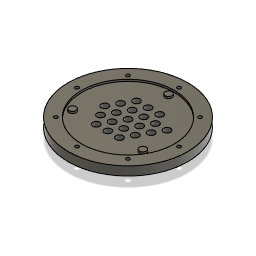
Feed.Through.Adapter (Autodesk Fusion 360 design; units mm, degrees)
Autodesk Fusion 360 part; units mm, degrees
note: some values were not read from the file. Chosen so that the rebuilt part matches the saved one: which bodies a step acts on.
sketch "Active.Area" plane through (0, 0, 0) normal (0, 1, 0) x (1, 0, 0)
  circle A0 centre (0, 0) radius 30
  circle A1 centre (0, 0) radius 40 construction
  circle A2 centre (0, -35) radius 3.175 construction
  circle A3 centre (30.3109, 17.5) radius 3.175 construction
  circle A4 centre (-30.3109, 17.5) radius 3.175 construction
  dimension "d1" = 60
  dimension "d2" = 80
  dimension "d4" = 6.35
  dimension "d6" = 360
  constraint coincident A0.centre A1.centre
  constraint concentric A0 A1
  measures "d1" diameter of A0
  measures "d2" diameter of A1
  measures "d4" diameter of A2
sketch "Feed.Through.Adapter.B" plane through (0, 0, 0) normal (0, 1, 0) x (1, 0, 0)
  circle A0 centre (0, 0) radius 34
  circle A1 centre (0, 0) radius 32 construction
  circle A2 centre (0, 32) radius 1
  circle A3 centre (-27.7128, -16) radius 1
  circle A4 centre (27.7128, -16) radius 1
  circle A5 centre (0, 0) radius 30 construction
  dimension "d7" = 68
  dimension "d8" = 64
  dimension "d9" = 2
  dimension "d11" = 360
  dimension "d12" = 60
  constraint coincident A0.centre A1.centre
  constraint concentric A0 A1
  constraint concentric A1 A5
  measures "d7" diameter of A0
  measures "d8" diameter of A1
  measures "d9" diameter of A2
  measures "d12" diameter of A5
sketch "Holes/Cuts" plane through (0, 0, 0) normal (0, 1, 0) x (1, 0, 0)
  circle A0 centre (0, 0) radius 30 construction
  circle A1 centre (0, 0) radius 3
  circle A2 centre (10, 0) radius 3
  circle A3 centre (5, 8.6603) radius 3
  circle A4 centre (-5, 8.6603) radius 3
  circle A5 centre (-10, 0) radius 3
  circle A6 centre (-5, -8.6603) radius 3
  circle A7 centre (5, -8.6603) radius 3
  circle A8 centre (15, 8.6603) radius 3
  circle A9 centre (0, 17.3205) radius 3
  circle A10 centre (-15, 8.6603) radius 3
  circle A11 centre (-15, -8.6603) radius 3
  circle A12 centre (0, -17.3205) radius 3
  circle A13 centre (15, -8.6603) radius 3
  circle A14 centre (20, 0) radius 3
  circle A15 centre (10, 17.3205) radius 3
  circle A16 centre (-10, 17.3205) radius 3
  circle A17 centre (-20, 0) radius 3
  circle A18 centre (-10, -17.3205) radius 3
  circle A19 centre (10, -17.3205) radius 3
  circle A20 centre (25, 8.6603) radius 3
  circle A21 centre (0, 0) radius 31
  circle A22 centre (0, 0) radius 40
  circle A23 centre (20, 0) radius 0.5
  circle A24 centre (10, 0) radius 0.5
  circle A25 centre (0, 0) radius 0.5
  circle A26 centre (15, -8.6603) radius 0.5
  circle A27 centre (5, 8.6603) radius 0.5
  circle A28 centre (10, 17.3205) radius 0.5
  circle A29 centre (15, 8.6603) radius 0.5
  circle A30 centre (-5, 8.6603) radius 0.5
  circle A31 centre (-10, 17.3205) radius 0.5
  circle A32 centre (0, 17.3205) radius 0.5
  circle A33 centre (-10, 0) radius 0.5
  circle A34 centre (-20, 0) radius 0.5
  circle A35 centre (-15, 8.6603) radius 0.5
  circle A36 centre (-5, -8.6603) radius 0.5
  circle A37 centre (-10, -17.3205) radius 0.5
  circle A38 centre (-15, -8.6603) radius 0.5
  circle A39 centre (5, -8.6603) radius 0.5
  circle A40 centre (10, -17.3205) radius 0.5
  circle A41 centre (0, -17.3205) radius 0.5
  circle A42 centre (25, 8.6603) radius 0.5
  dimension "d39" = 6
  dimension "d52" = 62
  dimension "d112" = 80
  dimension "d179" = 1
  dimension "d180" = 1
  dimension "d181" = 1
  dimension "d182" = 1
  dimension "d184" = 360
  dimension "d185" = 1
  constraint coincident A0.centre A1.centre
  constraint concentric A1 A22
  constraint concentric A14 A23
  constraint concentric A2 A24
  constraint concentric A0 A25
  constraint concentric A20 A42
  measures "d39" diameter of A1
  measures "d52" diameter of A21
  measures "d112" diameter of A22
  measures "d179" diameter of A23
  measures "d180" diameter of A24
  measures "d181" diameter of A25
  measures "d182" diameter of A26
  measures "d185" diameter of A42
extrude "Extrude1" add sketch "Feed.Through.Adapter.B" along normal blind 1.6 contours A2 | A3 | A4 makes body 1 at (-28.6343, 1.0667, 16.3884) makes body 2 at (0.9215, 1.0667, -32.3884) makes body 3 at (28.7078, 1.0667, 16.0996)
extrude "Extrude2" add sketch "Feed.Through.Adapter.B" along normal blind 6 from surface at 1.6 separate body makes body 4
extrude "Extrude3" cut sketch "Holes/Cuts" along normal blind 13 contours A1 | A2 | A3 | A4 | A5 | A6 | A7 | A8 | A9 | A10 | A11 | A12 | A13 | A14 | A15 | A16 | A17 | A18 | A19 | A20 | A23 | A24 | A25 | A26 | A27 | A28 | A29 | A30 | A31 | A32 | A33 | A34 | A35 | A36 | A37 | A38 | A39 | A40 | A41 | A42 bodies 4
extrude "Extrude4" add 3 faces at (27.094, 1.6, 16.2429) (0.3074, 1.6, -31.9503) (-27.1389, 1.6, 15.7236) along direction (0, 1, 0) blind 6 on bodies 1 2 3 bodies 3 1 2 4
sketch "Gasket.Cuts" plane through (0, 0, 0) normal (0, 1, 0) x (1, 0, 0)
  circle A0 centre (0, 0) radius 34
  circle A1 centre (0, 0) radius 33
  circle A2 centre (0, 0) radius 40
  circle A3 centre (0, 0) radius 36 construction
  circle A4 centre (0, 0) radius 35.5
  circle A5 centre (0, 0) radius 36.5
  dimension "d62" = 68
  dimension "d63" = 66
  dimension "d87" = 80
  dimension "d89" = 72
  dimension "d92" = 71
  dimension "d93" = 73
  constraint coincident A0.centre A1.centre
  constraint concentric A0 A2
  constraint concentric A1 A3
  constraint concentric A0 A4
  constraint concentric A0 A5
  measures "d62" diameter of A0
  measures "d63" diameter of A1
  measures "d87" diameter of A2
  measures "d89" diameter of A3
  measures "d92" diameter of A4
  measures "d93" diameter of A5
move_body "Move1" bodies 3 to x (1, 0, 0) y (0, 1, 0) z (0, 0, 1) at (0, -1.6, 0)
extrude "Extrude5" cut sketch "Gasket.Cuts" along normal blind 1 from surface at 3 contours A0 bodies 3
extrude "Extrude6" add 1 faces at (20.4746, 6, -17.2349) along direction (0, 1, 0) blind 1 on bodies 3 bodies 3
sketch "Feed.Through.Adapter.A" plane through (0, 0, 0) normal (0, 1, 0) x (1, 0, 0)
  circle A0 centre (0, 0) radius 40
  circle A1 centre (0, 0) radius 35 construction
  circle A2 centre (0, 35) radius 3
  circle A3 centre (-30.3109, -17.5) radius 3
  circle A4 centre (30.3109, -17.5) radius 3
  circle A5 centre (0, 0) radius 30 construction
  dimension "d69" = 80
  dimension "d70" = 70
  dimension "d71" = 6
  dimension "d73" = 360
  dimension "d74" = 60
  constraint coincident A0.centre A1.centre
  constraint coincident A1 A2.centre
  constraint concentric A0 A5
  measures "d69" diameter of A0
  measures "d70" diameter of A1
  measures "d71" diameter of A2
  measures "d74" diameter of A5
extrude "Extrude7" add sketch "Feed.Through.Adapter.A" along normal blind 5 from surface at 7 contours A0 | A2 | A3 | A4 bodies 3
extrude "Extrude8" add sketch "Feed.Through.Adapter.A" along normal blind 1.6 from surface at 13 separate body contours A2 | A3 | A4 makes body 5 at (33.296, 13.5333, 17.7987) makes body 6 at (-27.3258, 13.5333, 17.7987) makes body 7 at (2.9851, 13.5333, -34.7013)
extrude "Extrude9" add 1 faces at (9.4847, 12, 14.2223) along direction (0, 1, 0) blind 1 on bodies 3 bodies 3 5 6 7
extrude "Extrude10" cut 20 faces at (-19.6428, 7, 1.0398) (-8.4209, 7, -0.8733) (-15.0747, 7, 7.7957) (-5.1323, 7, 8.0449) (-11.5569, 7, 16.7572) (0.6235, 7, 18.4004) (8.7538, 7, 17.5489) (5.5984, 7, 8.0449) (16.1731, 7, 7.9138) (9.3572, 7, -1.0398) (1.2818, 7, 1.0989) (18.366, 7, -0.8804) (14.9253, 7, -9.5248) (4.8677, 7, -9.2756) (-4.8548, 7, -9.3845) (-13.3084, 7, -8.0321) (-10.7729, 7, -16.5387) (0.6916, 7, -17.819) (9.5, 7, -18.1865) (25.3505, 7, -9.5263) along direction (0, 1, 0) blind 25 on bodies 3 bodies 3
extrude "Extrude11" cut sketch "Gasket.Cuts" along normal blind 1 from surface at 7 contours A5 bodies 3
sketch "Screw.Size" plane through (0, 0, 0) normal (0, 1, 0) x (1, 0, 0)
  circle A0 centre (0, 0) radius 40
  circle A1 centre (0, 0) radius 51.5
  circle A2 centre (0, 0) radius 36.5 construction
  line L0 (0.0005, -36.5) -> (0.0005, -51.5) construction
  line L1 (0.0005, -36.5) -> (0.0005, -44) construction
  circle A3 centre (0, 0) radius 44 construction
  circle A4 centre (0.0005, -44) radius 1.5
  circle A5 centre (31.1131, -31.1123) radius 1.5
  circle A6 centre (44, 0.0005) radius 1.5
  circle A7 centre (31.1123, 31.1131) radius 1.5
  circle A8 centre (-0.0005, 44) radius 1.5
  circle A9 centre (-31.1131, 31.1123) radius 1.5
  circle A10 centre (-44, -0.0005) radius 1.5
  circle A11 centre (-31.1123, -31.1131) radius 1.5
  dimension "d97" = 80
  dimension "d103" = 103
  dimension "d104" = 73
  dimension "d105" = 7.5
  dimension "d106" = 3
  dimension "d108" = 360
  constraint coincident A0.centre A1.centre
  constraint concentric A0 A1
  constraint coincident A2 L0.start
  constraint coincident A1 L0.end
  constraint vertical L0
  constraint parallel L0 L1
  constraint concentric A1 A3
  constraint coincident L1.end A3
  constraint coincident L1.end A4.centre
  measures "d97" diameter of A0
  measures "d103" diameter of A1
  measures "d104" diameter of A2
  measures "d105" distance of L0.start L1.end
  measures "d106" diameter of A4
extrude "Extrude12" add sketch "Screw.Size" along normal blind 6 from surface at 7 bodies 3
extrude "Extrude13" add sketch "Screw.Size" along normal blind 1.6 from surface at 13 bodies 3
extrude "Extrude14" add sketch "Feed.Through.Adapter.B" against normal blind 1.6 separate body makes body 8
extrude "Extrude15" add sketch "Feed.Through.Adapter.A" along normal blind 1.6 from surface at 13 separate body makes body 9
extrude "Extrude16" cut sketch "Active.Area" along normal blind 4 from surface at 14.5 bodies 9
sketch "Sketch7" plane through (0, 0, 0) normal (0, 1, 0) x (1, 0, 0)
  circle A0 centre (0, 0) radius 30 construction
  circle A1 centre (0, 0) radius 40 construction
  circle A2 centre (0, 0) radius 30
  line L0 (3.18, 2.4133) -> (0.5, 3.9606)
  line L1 (-0.5, 3.9606) -> (-3.18, 2.4133)
  line L2 (-3.68, 1.5473) -> (-3.68, -1.5473)
  line L3 (-3.18, -2.4133) -> (-0.5, -3.9606)
  line L4 (0.5, -3.9606) -> (3.18, -2.4133)
  line L5 (3.68, -1.5473) -> (3.68, 1.5473)
  line L6 (-6.82, 2.4133) -> (-9.5, 3.9606)
  line L7 (-10.5, 3.9606) -> (-13.18, 2.4133)
  line L8 (-13.68, 1.5473) -> (-13.68, -1.5473)
  line L9 (-13.18, -2.4133) -> (-10.5, -3.9606)
  line L10 (-9.5, -3.9606) -> (-6.82, -2.4133)
  line L11 (-6.32, -1.5473) -> (-6.32, 1.5473)
  line L12 (-16.82, 2.4133) -> (-19.5, 3.9606)
  line L13 (-20.5, 3.9606) -> (-23.18, 2.4133)
  line L14 (-23.68, 1.5473) -> (-23.68, -1.5473)
  line L15 (-23.18, -2.4133) -> (-20.5, -3.9606)
  line L16 (-19.5, -3.9606) -> (-16.82, -2.4133)
  line L17 (-16.32, -1.5473) -> (-16.32, 1.5473)
  line L18 (-11.82, -6.2469) -> (-14.5, -4.6996)
  line L19 (-15.5, -4.6996) -> (-18.18, -6.2469)
  line L20 (-18.68, -7.113) -> (-18.68, -10.2076)
  line L21 (-18.18, -11.0736) -> (-15.5, -12.6209)
  line L22 (-14.5, -12.6209) -> (-11.82, -11.0736)
  line L23 (-11.32, -10.2076) -> (-11.32, -7.113)
  arc A3 (0.5, 3.9606) -> (-0.5, 3.9606) centre (0, 3.0946) ccw
  arc A4 (3.68, 1.5473) -> (3.18, 2.4133) centre (2.68, 1.5473) ccw
  arc A5 (3.18, -2.4133) -> (3.68, -1.5473) centre (2.68, -1.5473) ccw
  arc A6 (-0.5, -3.9606) -> (0.5, -3.9606) centre (0, -3.0946) ccw
  arc A7 (-3.68, -1.5473) -> (-3.18, -2.4133) centre (-2.68, -1.5473) ccw
  arc A8 (-3.18, 2.4133) -> (-3.68, 1.5473) centre (-2.68, 1.5473) ccw
  arc A9 (-6.32, 1.5473) -> (-6.82, 2.4133) centre (-7.32, 1.5473) ccw
  arc A10 (-9.5, 3.9606) -> (-10.5, 3.9606) centre (-10, 3.0946) ccw
  arc A11 (-13.18, 2.4133) -> (-13.68, 1.5473) centre (-12.68, 1.5473) ccw
  arc A12 (-13.68, -1.5473) -> (-13.18, -2.4133) centre (-12.68, -1.5473) ccw
  arc A13 (-10.5, -3.9606) -> (-9.5, -3.9606) centre (-10, -3.0946) ccw
  arc A14 (-6.82, -2.4133) -> (-6.32, -1.5473) centre (-7.32, -1.5473) ccw
  arc A15 (-20.5, -3.9606) -> (-19.5, -3.9606) centre (-20, -3.0946) ccw
  arc A16 (-16.82, -2.4133) -> (-16.32, -1.5473) centre (-17.32, -1.5473) ccw
  arc A17 (-16.32, 1.5473) -> (-16.82, 2.4133) centre (-17.32, 1.5473) ccw
  arc A18 (-19.5, 3.9606) -> (-20.5, 3.9606) centre (-20, 3.0946) ccw
  arc A19 (-23.18, 2.4133) -> (-23.68, 1.5473) centre (-22.68, 1.5473) ccw
  arc A20 (-23.68, -1.5473) -> (-23.18, -2.4133) centre (-22.68, -1.5473) ccw
  arc A21 (-18.18, -6.2469) -> (-18.68, -7.113) centre (-17.68, -7.113) ccw
  arc A22 (-14.5, -4.6996) -> (-15.5, -4.6996) centre (-15, -5.5657) ccw
  arc A23 (-11.32, -7.113) -> (-11.82, -6.2469) centre (-12.32, -7.113) ccw
  arc A24 (-11.82, -11.0736) -> (-11.32, -10.2076) centre (-12.32, -10.2076) ccw
  arc A25 (-15.5, -12.6209) -> (-14.5, -12.6209) centre (-15, -11.7549) ccw
  arc A26 (-18.68, -10.2076) -> (-18.18, -11.0736) centre (-17.68, -10.2076) ccw
  arc A27 (-5.5, -12.6209) -> (-4.5, -12.6209) centre (-5, -11.7549) ccw
  line L24 (-8.18, -11.0736) -> (-5.5, -12.6209)
  line L25 (-1.32, -10.2076) -> (-1.32, -7.113)
  arc A28 (-1.32, -7.113) -> (-1.82, -6.2469) centre (-2.32, -7.113) ccw
  arc A29 (-1.82, -11.0736) -> (-1.32, -10.2076) centre (-2.32, -10.2076) ccw
  line L26 (-8.68, -7.113) -> (-8.68, -10.2076)
  arc A30 (-8.68, -10.2076) -> (-8.18, -11.0736) centre (-7.68, -10.2076) ccw
  arc A31 (-4.5, -4.6996) -> (-5.5, -4.6996) centre (-5, -5.5657) ccw
  line L27 (-4.5, -12.6209) -> (-1.82, -11.0736)
  line L28 (-5.5, -4.6996) -> (-8.18, -6.2469)
  arc A32 (-8.18, -6.2469) -> (-8.68, -7.113) centre (-7.68, -7.113) ccw
  line L29 (-1.82, -6.2469) -> (-4.5, -4.6996)
  arc A33 (8.18, -11.0736) -> (8.68, -10.2076) centre (7.68, -10.2076) ccw
  line L30 (5.5, -12.6209) -> (8.18, -11.0736)
  line L31 (8.18, -6.2469) -> (5.5, -4.6996)
  arc A34 (5.5, -4.6996) -> (4.5, -4.6996) centre (5, -5.5657) ccw
  arc A35 (8.68, -7.113) -> (8.18, -6.2469) centre (7.68, -7.113) ccw
  line L32 (1.82, -11.0736) -> (4.5, -12.6209)
  arc A36 (4.5, -12.6209) -> (5.5, -12.6209) centre (5, -11.7549) ccw
  arc A37 (1.82, -6.2469) -> (1.32, -7.113) centre (2.32, -7.113) ccw
  line L33 (8.68, -10.2076) -> (8.68, -7.113)
  line L34 (1.32, -7.113) -> (1.32, -10.2076)
  arc A38 (1.32, -10.2076) -> (1.82, -11.0736) centre (2.32, -10.2076) ccw
  line L35 (4.5, -4.6996) -> (1.82, -6.2469)
  arc A39 (13.68, 1.5473) -> (13.18, 2.4133) centre (12.68, 1.5473) ccw
  line L36 (13.68, -1.5473) -> (13.68, 1.5473)
  line L37 (9.5, 3.9606) -> (6.82, 2.4133)
  arc A40 (6.82, 2.4133) -> (6.32, 1.5473) centre (7.32, 1.5473) ccw
  arc A41 (10.5, 3.9606) -> (9.5, 3.9606) centre (10, 3.0946) ccw
  line L38 (10.5, -3.9606) -> (13.18, -2.4133)
  arc A42 (13.18, -2.4133) -> (13.68, -1.5473) centre (12.68, -1.5473) ccw
  arc A43 (6.32, -1.5473) -> (6.82, -2.4133) centre (7.32, -1.5473) ccw
  line L39 (13.18, 2.4133) -> (10.5, 3.9606)
  line L40 (6.82, -2.4133) -> (9.5, -3.9606)
  arc A44 (9.5, -3.9606) -> (10.5, -3.9606) centre (10, -3.0946) ccw
  line L41 (6.32, 1.5473) -> (6.32, -1.5473)
  arc A45 (5.5, 12.6209) -> (4.5, 12.6209) centre (5, 11.7549) ccw
  line L42 (8.18, 11.0736) -> (5.5, 12.6209)
  line L43 (1.32, 10.2076) -> (1.32, 7.113)
  arc A46 (1.32, 7.113) -> (1.82, 6.2469) centre (2.32, 7.113) ccw
  arc A47 (1.82, 11.0736) -> (1.32, 10.2076) centre (2.32, 10.2076) ccw
  line L44 (8.68, 7.113) -> (8.68, 10.2076)
  arc A48 (8.68, 10.2076) -> (8.18, 11.0736) centre (7.68, 10.2076) ccw
  arc A49 (4.5, 4.6996) -> (5.5, 4.6996) centre (5, 5.5657) ccw
  line L45 (4.5, 12.6209) -> (1.82, 11.0736)
  line L46 (5.5, 4.6996) -> (8.18, 6.2469)
  arc A50 (8.18, 6.2469) -> (8.68, 7.113) centre (7.68, 7.113) ccw
  line L47 (1.82, 6.2469) -> (4.5, 4.6996)
  arc A51 (-8.18, 11.0736) -> (-8.68, 10.2076) centre (-7.68, 10.2076) ccw
  line L48 (-5.5, 12.6209) -> (-8.18, 11.0736)
  line L49 (-8.18, 6.2469) -> (-5.5, 4.6996)
  arc A52 (-5.5, 4.6996) -> (-4.5, 4.6996) centre (-5, 5.5657) ccw
  arc A53 (-8.68, 7.113) -> (-8.18, 6.2469) centre (-7.68, 7.113) ccw
  line L50 (-1.82, 11.0736) -> (-4.5, 12.6209)
  arc A54 (-4.5, 12.6209) -> (-5.5, 12.6209) centre (-5, 11.7549) ccw
  arc A55 (-1.82, 6.2469) -> (-1.32, 7.113) centre (-2.32, 7.113) ccw
  line L51 (-8.68, 10.2076) -> (-8.68, 7.113)
  line L52 (-1.32, 7.113) -> (-1.32, 10.2076)
  arc A56 (-1.32, 10.2076) -> (-1.82, 11.0736) centre (-2.32, 10.2076) ccw
  line L53 (-4.5, 4.6996) -> (-1.82, 6.2469)
  arc A57 (-3.18, -14.9072) -> (-3.68, -15.7732) centre (-2.68, -15.7732) ccw
  line L54 (-0.5, -13.3599) -> (-3.18, -14.9072)
  line L55 (-3.68, -15.7732) -> (-3.68, -18.8678)
  arc A58 (-3.68, -18.8678) -> (-3.18, -19.7338) centre (-2.68, -18.8678) ccw
  line L56 (-3.18, -19.7338) -> (-0.5, -21.2811)
  arc A59 (-0.5, -21.2811) -> (0.5, -21.2811) centre (0, -20.4151) ccw
  line L57 (0.5, -21.2811) -> (3.18, -19.7338)
  arc A60 (3.18, -19.7338) -> (3.68, -18.8678) centre (2.68, -18.8678) ccw
  line L58 (3.68, -18.8678) -> (3.68, -15.7732)
  arc A61 (3.68, -15.7732) -> (3.18, -14.9072) centre (2.68, -15.7732) ccw
  line L59 (3.18, -14.9072) -> (0.5, -13.3599)
  arc A62 (0.5, -13.3599) -> (-0.5, -13.3599) centre (0, -14.2259) ccw
  arc A63 (11.32, -10.2076) -> (11.82, -11.0736) centre (12.32, -10.2076) ccw
  line L60 (11.32, -7.113) -> (11.32, -10.2076)
  line L61 (11.82, -11.0736) -> (14.5, -12.6209)
  arc A64 (14.5, -12.6209) -> (15.5, -12.6209) centre (15, -11.7549) ccw
  line L62 (15.5, -12.6209) -> (18.18, -11.0736)
  arc A65 (18.18, -11.0736) -> (18.68, -10.2076) centre (17.68, -10.2076) ccw
  line L63 (18.68, -10.2076) -> (18.68, -7.113)
  arc A66 (18.68, -7.113) -> (18.18, -6.2469) centre (17.68, -7.113) ccw
  line L64 (18.18, -6.2469) -> (15.5, -4.6996)
  arc A67 (15.5, -4.6996) -> (14.5, -4.6996) centre (15, -5.5657) ccw
  line L65 (14.5, -4.6996) -> (11.82, -6.2469)
  arc A68 (11.82, -6.2469) -> (11.32, -7.113) centre (12.32, -7.113) ccw
  arc A69 (14.5, 4.6996) -> (15.5, 4.6996) centre (15, 5.5657) ccw
  line L66 (11.82, 6.2469) -> (14.5, 4.6996)
  line L67 (15.5, 4.6996) -> (18.18, 6.2469)
  arc A70 (18.18, 6.2469) -> (18.68, 7.113) centre (17.68, 7.113) ccw
  line L68 (18.68, 7.113) -> (18.68, 10.2076)
  arc A71 (18.68, 10.2076) -> (18.18, 11.0736) centre (17.68, 10.2076) ccw
  line L69 (18.18, 11.0736) -> (15.5, 12.6209)
  arc A72 (15.5, 12.6209) -> (14.5, 12.6209) centre (15, 11.7549) ccw
  line L70 (14.5, 12.6209) -> (11.82, 11.0736)
  arc A73 (11.82, 11.0736) -> (11.32, 10.2076) centre (12.32, 10.2076) ccw
  line L71 (11.32, 10.2076) -> (11.32, 7.113)
  arc A74 (11.32, 7.113) -> (11.82, 6.2469) centre (12.32, 7.113) ccw
  arc A75 (3.18, 14.9072) -> (3.68, 15.7732) centre (2.68, 15.7732) ccw
  line L72 (0.5, 13.3599) -> (3.18, 14.9072)
  line L73 (3.68, 15.7732) -> (3.68, 18.8678)
  arc A76 (3.68, 18.8678) -> (3.18, 19.7338) centre (2.68, 18.8678) ccw
  line L74 (3.18, 19.7338) -> (0.5, 21.2811)
  arc A77 (0.5, 21.2811) -> (-0.5, 21.2811) centre (0, 20.4151) ccw
  line L75 (-0.5, 21.2811) -> (-3.18, 19.7338)
  arc A78 (-3.18, 19.7338) -> (-3.68, 18.8678) centre (-2.68, 18.8678) ccw
  line L76 (-3.68, 18.8678) -> (-3.68, 15.7732)
  arc A79 (-3.68, 15.7732) -> (-3.18, 14.9072) centre (-2.68, 15.7732) ccw
  line L77 (-3.18, 14.9072) -> (-0.5, 13.3599)
  arc A80 (-0.5, 13.3599) -> (0.5, 13.3599) centre (0, 14.2259) ccw
  arc A81 (-11.32, 10.2076) -> (-11.82, 11.0736) centre (-12.32, 10.2076) ccw
  line L78 (-11.32, 7.113) -> (-11.32, 10.2076)
  line L79 (-11.82, 11.0736) -> (-14.5, 12.6209)
  arc A82 (-14.5, 12.6209) -> (-15.5, 12.6209) centre (-15, 11.7549) ccw
  line L80 (-15.5, 12.6209) -> (-18.18, 11.0736)
  arc A83 (-18.18, 11.0736) -> (-18.68, 10.2076) centre (-17.68, 10.2076) ccw
  line L81 (-18.68, 10.2076) -> (-18.68, 7.113)
  arc A84 (-18.68, 7.113) -> (-18.18, 6.2469) centre (-17.68, 7.113) ccw
  line L82 (-18.18, 6.2469) -> (-15.5, 4.6996)
  arc A85 (-15.5, 4.6996) -> (-14.5, 4.6996) centre (-15, 5.5657) ccw
  line L83 (-14.5, 4.6996) -> (-11.82, 6.2469)
  arc A86 (-11.82, 6.2469) -> (-11.32, 7.113) centre (-12.32, 7.113) ccw
  line L84 (-6.32, -18.8678) -> (-6.32, -15.7732)
  line L85 (-13.68, -15.7732) -> (-13.68, -18.8678)
  line L86 (-10.5, -13.3599) -> (-13.18, -14.9072)
  arc A87 (-6.32, -15.7732) -> (-6.82, -14.9072) centre (-7.32, -15.7732) ccw
  arc A88 (-13.18, -14.9072) -> (-13.68, -15.7732) centre (-12.68, -15.7732) ccw
  arc A89 (-10.5, -21.2811) -> (-9.5, -21.2811) centre (-10, -20.4151) ccw
  arc A90 (-6.82, -19.7338) -> (-6.32, -18.8678) centre (-7.32, -18.8678) ccw
  line L87 (-6.82, -14.9072) -> (-9.5, -13.3599)
  arc A91 (-9.5, -13.3599) -> (-10.5, -13.3599) centre (-10, -14.2259) ccw
  line L88 (-9.5, -21.2811) -> (-6.82, -19.7338)
  arc A92 (-13.68, -18.8678) -> (-13.18, -19.7338) centre (-12.68, -18.8678) ccw
  line L89 (-13.18, -19.7338) -> (-10.5, -21.2811)
  line L90 (13.18, -14.9072) -> (10.5, -13.3599)
  line L91 (6.82, -19.7338) -> (9.5, -21.2811)
  line L92 (6.32, -15.7732) -> (6.32, -18.8678)
  arc A93 (10.5, -13.3599) -> (9.5, -13.3599) centre (10, -14.2259) ccw
  arc A94 (6.32, -18.8678) -> (6.82, -19.7338) centre (7.32, -18.8678) ccw
  arc A95 (13.18, -19.7338) -> (13.68, -18.8678) centre (12.68, -18.8678) ccw
  arc A96 (13.68, -15.7732) -> (13.18, -14.9072) centre (12.68, -15.7732) ccw
  line L93 (9.5, -13.3599) -> (6.82, -14.9072)
  arc A97 (6.82, -14.9072) -> (6.32, -15.7732) centre (7.32, -15.7732) ccw
  line L94 (13.68, -18.8678) -> (13.68, -15.7732)
  arc A98 (9.5, -21.2811) -> (10.5, -21.2811) centre (10, -20.4151) ccw
  line L95 (10.5, -21.2811) -> (13.18, -19.7338)
  line L96 (19.5, 3.9606) -> (16.82, 2.4133)
  line L97 (20.5, -3.9606) -> (23.18, -2.4133)
  line L98 (16.82, -2.4133) -> (19.5, -3.9606)
  arc A99 (16.82, 2.4133) -> (16.32, 1.5473) centre (17.32, 1.5473) ccw
  arc A100 (19.5, -3.9606) -> (20.5, -3.9606) centre (20, -3.0946) ccw
  arc A101 (23.68, 1.5473) -> (23.18, 2.4133) centre (22.68, 1.5473) ccw
  arc A102 (20.5, 3.9606) -> (19.5, 3.9606) centre (20, 3.0946) ccw
  line L99 (16.32, 1.5473) -> (16.32, -1.5473)
  arc A103 (16.32, -1.5473) -> (16.82, -2.4133) centre (17.32, -1.5473) ccw
  line L100 (23.18, 2.4133) -> (20.5, 3.9606)
  arc A104 (23.18, -2.4133) -> (23.68, -1.5473) centre (22.68, -1.5473) ccw
  line L101 (23.68, -1.5473) -> (23.68, 1.5473)
  line L102 (6.32, 18.8678) -> (6.32, 15.7732)
  line L103 (13.68, 15.7732) -> (13.68, 18.8678)
  line L104 (10.5, 13.3599) -> (13.18, 14.9072)
  arc A105 (6.32, 15.7732) -> (6.82, 14.9072) centre (7.32, 15.7732) ccw
  arc A106 (13.18, 14.9072) -> (13.68, 15.7732) centre (12.68, 15.7732) ccw
  arc A107 (10.5, 21.2811) -> (9.5, 21.2811) centre (10, 20.4151) ccw
  arc A108 (6.82, 19.7338) -> (6.32, 18.8678) centre (7.32, 18.8678) ccw
  line L105 (6.82, 14.9072) -> (9.5, 13.3599)
  arc A109 (9.5, 13.3599) -> (10.5, 13.3599) centre (10, 14.2259) ccw
  line L106 (9.5, 21.2811) -> (6.82, 19.7338)
  arc A110 (13.68, 18.8678) -> (13.18, 19.7338) centre (12.68, 18.8678) ccw
  line L107 (13.18, 19.7338) -> (10.5, 21.2811)
  line L108 (-13.18, 14.9072) -> (-10.5, 13.3599)
  line L109 (-6.82, 19.7338) -> (-9.5, 21.2811)
  line L110 (-6.32, 15.7732) -> (-6.32, 18.8678)
  arc A111 (-10.5, 13.3599) -> (-9.5, 13.3599) centre (-10, 14.2259) ccw
  arc A112 (-6.32, 18.8678) -> (-6.82, 19.7338) centre (-7.32, 18.8678) ccw
  arc A113 (-13.18, 19.7338) -> (-13.68, 18.8678) centre (-12.68, 18.8678) ccw
  arc A114 (-13.68, 15.7732) -> (-13.18, 14.9072) centre (-12.68, 15.7732) ccw
  line L111 (-9.5, 13.3599) -> (-6.82, 14.9072)
  arc A115 (-6.82, 14.9072) -> (-6.32, 15.7732) centre (-7.32, 15.7732) ccw
  line L112 (-13.68, 18.8678) -> (-13.68, 15.7732)
  arc A116 (-9.5, 21.2811) -> (-10.5, 21.2811) centre (-10, 20.4151) ccw
  line L113 (-10.5, 21.2811) -> (-13.18, 19.7338)
  point P0 (-20, 0)
  point P1 (-10, 0)
  point P2 (-20, 0)
  point P3 (-15, -8.6603)
  point P4 (-5, -8.6603)
  point P5 (5, -8.6603)
  point P6 (10, 0)
  point P7 (5, 8.6603)
  point P8 (-5, 8.6603)
  point P9 (-10, -17.3205)
  point P10 (-10, -17.3205)
  point P11 (10, -17.3205)
  point P12 (10, -17.3205)
  point P13 (20, 0)
  point P14 (20, 0)
  point P15 (10, 17.3205)
  point P16 (10, 17.3205)
  point P17 (-10, 17.3205)
  point P18 (-10, 17.3205)
  dimension "d172" = 1
  dimension "d174" = 360
  dimension "d176" = 360
  dimension "d178" = 360
  constraint coincident A0.centre A1.centre
  constraint concentric A0 A1
  constraint coincident P2 P0
  constraint tangent L0 A3
  constraint tangent L1 A3
  constraint tangent L0 A4
  constraint tangent L5 A4
  constraint equal A3 A4
  constraint tangent L4 A5
  constraint tangent L5 A5
  constraint equal A3 A5
  constraint tangent L3 A6
  constraint tangent L4 A6
  constraint equal A3 A6
  constraint tangent L2 A7
  constraint tangent L3 A7
  constraint equal A3 A7
  constraint tangent L1 A8
  constraint tangent L2 A8
  constraint equal A3 A8
  constraint tangent L6 A9
  constraint tangent L11 A9
  constraint equal A3 A9
  constraint tangent L6 A10
  constraint tangent L7 A10
  constraint equal A3 A10
  constraint tangent L7 A11
  constraint tangent L8 A11
  constraint equal A3 A11
  constraint tangent L8 A12
  constraint tangent L9 A12
  constraint equal A3 A12
  constraint tangent L9 A13
  constraint tangent L10 A13
  constraint equal A3 A13
  constraint tangent L10 A14
  constraint tangent L11 A14
  constraint equal A3 A14
  constraint tangent L15 A15
  constraint tangent L16 A15
  constraint equal A3 A15
  constraint tangent L16 A16
  constraint tangent L17 A16
  constraint equal A3 A16
  constraint tangent L12 A17
  constraint tangent L17 A17
  constraint equal A3 A17
  constraint tangent L12 A18
  constraint tangent L13 A18
  constraint equal A3 A18
  constraint tangent L13 A19
  constraint tangent L14 A19
  constraint equal A3 A19
  constraint tangent L14 A20
  constraint tangent L15 A20
  constraint equal A3 A20
  constraint tangent L19 A21
  constraint tangent L20 A21
  constraint equal A3 A21
  constraint tangent L18 A22
  constraint tangent L19 A22
  constraint equal A3 A22
  constraint tangent L18 A23
  constraint tangent L23 A23
  constraint equal A3 A23
  constraint tangent L22 A24
  constraint tangent L23 A24
  constraint equal A3 A24
  constraint tangent L21 A25
  constraint tangent L22 A25
  constraint equal A3 A25
  constraint tangent L20 A26
  constraint tangent L21 A26
  constraint equal A3 A26
  measures "d172" radius of A3
extrude "Extrude18" cut sketch "Holes/Cuts" along normal mid plane 58 contours A23 | A24 | A25 | A26 | A27 | A28 | A29 | A30 | A31 | A32 | A33 | A34 | A35 | A36 | A37 | A38 | A39 | A40 | A41 | A42 bodies 8 9
extrude "Extrude20" add sketch "Holes/Cuts" along normal blind 1.6 separate body contours A23 | A24 | A25 | A26 | A27 | A28 | A29 | A30 | A31 | A32 | A33 | A34 | A35 | A36 | A37 | A38 | A39 | A40 | A41 | A42 makes body 10 at (-10.4698, 1.0667, 17.1495) makes body 11 at (15.383, 1.0667, 8.3389) makes body 12 at (-9.5025, 1.0667, 0.0498) makes body 13 at (5.4975, 1.0667, -8.6105) makes body 14 at (-0.4607, 1.0667, -17.1263) makes body 15 at (9.5302, 1.0667, -17.4915) makes body 16 at (15.383, 1.0667, -8.9816) makes body 17 at (0.4975, 1.0667, 0.0498) makes body 18 at (5.4975, 1.0667, 8.71) makes body 19 at (-0.4607, 1.0667, 17.5147) makes body 20 at (-14.617, 1.0667, 8.3389) makes body 21 at (19.6509, 1.0667, -0.3579) makes body 22 at (-20.3491, 1.0667, -0.3579) makes body 23 at (-4.5025, 1.0667, -8.6105) makes body 24 at (-10.4698, 1.0667, -17.4915) makes body 25 at (-14.617, 1.0667, -8.9816) makes body 26 at (25.4607, 1.0667, -8.8545) makes body 27 at (10.4975, 1.0667, 0.0498) makes body 28 at (-4.5025, 1.0667, 8.71) makes body 29 at (9.5302, 1.0667, 17.1495)
move_body "Move2" bodies 10 22 19 20 18 29 23 24 25 26 27 28 16 21 11 12 13 14 15 17 to x (1, 0, 0) y (0, 1, 0) z (0, 0, 1) at (0, -1.6, 0)
extrude "Extrude21" add 20 faces at (19.8037, -1.6, 0.1134) (10.3208, -1.6, 0.1357) (14.7519, -1.6, 8.7399) (5.0774, -1.6, 8.8877) (10.1576, -1.6, 17.4419) (0.1277, -1.6, 17.5078) (-4.9662, -1.6, 8.7464) (-9.8424, -1.6, 17.4419) (-15.2481, -1.6, 8.7399) (-20.1963, -1.6, 0.1134) (-9.6792, -1.6, 0.1357) (0.4036, -1.6, 0.0491) (5.0774, -1.6, -8.4328) (-5.1104, -1.6, -8.585) (-15.2481, -1.6, -8.5806) (-9.8424, -1.6, -17.1991) (0.1277, -1.6, -17.1332) (10.1576, -1.6, -17.1991) (14.7519, -1.6, -8.5806) (24.8037, -1.6, -8.5469) along direction (0, -1, 0) blind 1.6 separate body on bodies 10 11 12 13 14 15 16 17 18 19 20 21 22 23 24 25 26 27 28 29 makes body 30 at (15.3986, -2.6667, -8.9622) makes body 31 at (-0.4607, -2.6667, -17.1263) makes body 32 at (-14.6014, -2.6667, -8.9622) makes body 33 at (5.4994, -2.6667, -8.6353) makes body 34 at (-9.5006, -2.6667, 0.0249) makes body 35 at (-14.6014, -2.6667, 8.3584) makes body 36 at (-4.5006, -2.6667, 8.6852) makes body 37 at (9.5302, -2.6667, 17.1495) makes body 38 at (15.3986, -2.6667, 8.3584) makes body 39 at (19.6509, -2.6667, -0.3579) makes body 40 at (10.4994, -2.6667, 0.0249) makes body 41 at (5.4994, -2.6667, 8.6852) makes body 42 at (-0.4607, -2.6667, 17.5147) makes body 43 at (-10.4698, -2.6667, 17.1495) makes body 44 at (-20.3491, -2.6667, -0.3579) makes body 45 at (0.4994, -2.6667, 0.0249) makes body 46 at (-4.5006, -2.6667, -8.6353) makes body 47 at (-10.4698, -2.6667, -17.4915) makes body 48 at (9.5302, -2.6667, -17.4915) makes body 49 at (25.4607, -2.6667, -8.8545)
move_body "Move3" bodies 30 44 45 32 31 37 33 40 36 38 35 41 42 34 39 46 47 49 48 43 to x (1, 0, 0) y (0, 1, 0) z (0, 0, 1) at (0, 16.2, 0)
sketch "Sketch8" plane through (0, 0, 0) normal (1, 0, 0) x (0, 0, -1)
  line L0 (0, 0) -> (-55, 0)
  line L1 (-55, 0) -> (-55, 25)
  line L2 (-55, 25) -> (0, 25)
  line L3 (0, 25) -> (0, 0)
  line L4 (-55, 0) -> (0, 0)
  line L5 (0, 0) -> (0, -25)
  line L6 (0, -25) -> (-55, -25)
  line L7 (-55, -25) -> (-55, 0)
  dimension "d196" = 55
  dimension "d197" = 25
  dimension "d198" = 25
  constraint horizontal L0
  constraint vertical L1
  constraint horizontal L2
  constraint vertical L3
  constraint coincident L0.start L3.end
  constraint horizontal L4
  constraint vertical L5
  constraint horizontal L6
  constraint vertical L7
  measures "d196" distance of L0.start L0.end
  measures "d197" distance of L0.start L2.end
  measures "d198" distance of L0.end L6.end
extrude "Extrude22" add sketch "Holes/Cuts" along normal blind 13 separate body contours A1 | A2 | A12 | A14 makes body 50 at (2.9851, 8.6667, 0.2987) makes body 51 at (12.9851, 8.6667, 0.2987) makes body 52 at (2.9851, 8.6667, 17.6192) makes body 53 at (22.9851, 8.6667, 0.2987)
extrude "Extrude19" [suppressed]
extrude "Extrude17" [suppressed]
named bodies: "Readout.Adapter", "Readout.PCB.B", "Readout.PCB.A"
